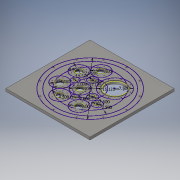
# Autodesk Inventor part: Top Plate
Saved by Autodesk Inventor 2018 (Build 220112000, 112)
## iProperties
Created: 2018-08-07
Part Number: Top Plate
Material: Stainless Steel, Austenitic
Document SubType Name: Modeling
Designer: freyja
Density: 8 g/cm^3
Appearance: Semi-Polished
Mass: 52241 g
Surface Area: 7917.75 cm^2
Volume: 6530.12 cm^3
Author: freyja
Autodesk Inventor part; units mm, degrees
ref_plane "YZ Plane" through (0, 0, 0) normal (1, 0, 0) x (0, 1, 0)
ref_plane "XZ Plane" through (0, 0, 0) normal (0, 1, 0) x (-1, 0, 0)
ref_plane "XY Plane" through (0, 0, 0) normal (0, 0, 1) x (1, 0, 0)
sketch "Sketch1" plane through (0, 0, 0) normal (0, 1, 0) x (-1, 0, 0)
  line L0 (304.8, 304.8) -> (-304.8, 304.8)
  line L1 (-304.8, 304.8) -> (-304.8, -304.8)
  line L2 (-304.8, -304.8) -> (304.8, -304.8)
  line L3 (304.8, -304.8) -> (304.8, 304.8)
  line L4 (304.8, 304.8) -> (-304.8, -304.8) construction
  line L5 (-304.8, 304.8) -> (304.8, -304.8) construction
  point P0 (0, 0)
  dimension "d0" = 609.6
  dimension "d1" = 609.6
  constraints: 12 end point, 2 midpoint, 2 parallel, 1 horizontal, 1 perpendicular
  measures "d0" distance of L2.end L1.end
  measures "d1" distance of L1.end L0.end
extrude "Extrusion1" add sketch "Sketch1" along normal blind 19.05
sketch "Sketch23" plane through (0, 19.05, 0) normal (0, 1, 0) x (1, 0, 0)
  circle A0 centre (0, 0) radius 273.05
  circle A1 centre (0, 0) radius 242.8875
  circle A2 centre (0, 0) radius 90.4875
  circle A3 centre (0, 0) radius 192.0875
  dimension "d167" = 546.1
  dimension "d168" = 485.775
  dimension "d292" = 180.975
  dimension "d293" = 384.175
  constraints: 4 centre point, 4 coincident
  measures "d167" diameter of A0
  measures "d168" diameter of A1
  measures "d292" diameter of A2
  measures "d293" diameter of A3
sketch "Sketch2" plane through (0, 19.05, 0) normal (0, 1, 0) x (1, 0, 0)
  line L0 (0, 0) -> (89.8026, 89.8026) construction
  line L1 (0, 0) -> (127, 0) construction
  circle A0 centre (89.8026, 89.8026) radius 118.745 construction
  circle A1 centre (89.8026, 89.8026) radius 66.675
  dimension "d4" = 127
  dimension "d5" = 45
  dimension "d6" = 237.49
  dimension "d7" = 133.35
  constraints: 4 end point, 2 centre point, 2 coincident, 1 equal length, 1 horizontal
  measures "d4" distance of L0.start L0.end
  measures "d5" angle of L1 L0
  measures "d6" diameter of A0
  measures "d7" diameter of A1
extrude "Extrusion2" cut sketch "Sketch2" against normal up to surface (19.05 mm away)
sketch "Sketch38" plane through (0, 19.05, 0) normal (0, 1, 0) x (1, 0, 0)
  circle A0 centre (89.8026, 89.8026) radius 66.675 projected
  circle A1 centre (89.8026, 89.8026) radius 71.247
  circle A2 centre (89.8026, 89.8026) radius 74.93
  point P0 (0, 0)
  dimension "d288" = 142.494
  dimension "d289" = 149.86
  constraints: 2 centre point, 2 coincident
  measures "d288" diameter of A1
  measures "d289" diameter of A2
extrude "Extrusion22" cut sketch "Sketch38" against normal blind 3.175 contours A2
sketch "Sketch3" plane through (0, 19.05, 0) normal (0, 1, 0) x (1, 0, 0)
  circle A0 centre (89.8026, 89.8026) radius 66.675 projected
  line L0 (89.8026, 89.8026) -> (169.5888, 56.754) construction
  line L1 (89.8026, 89.8026) -> (169.5888, 122.8511) construction
  line L2 (89.8026, 89.8026) -> (122.8511, 169.5888) construction
  line L3 (89.8026, 89.8026) -> (56.754, 169.5888) construction
  line L4 (89.8026, 89.8026) -> (10.0163, 122.8511) construction
  line L5 (89.8026, 89.8026) -> (10.0163, 56.754) construction
  line L6 (89.8026, 89.8026) -> (56.754, 10.0163) construction
  line L7 (89.8026, 89.8026) -> (122.8511, 10.0163) construction
  line L8 (89.8026, 89.8026) -> (136.7356, 70.3622) construction
  line L9 (89.8026, 89.8026) -> (140.6026, 89.8026) construction
  point P0 (0, 0)
  dimension "d10" = 86.36
  dimension "d14" = 360
  dimension "d408" = 50.8
  dimension "d409" = 22.5
  constraints: 20 end point, 2 coincident, 1 collinear, 1 equal length, 1 horizontal, 23 other
  measures "d10" distance of L0.start L0.end
  measures "d408" distance of L7.start L8.end
  measures "d409" angle of L8 L9
hole "Hole1" at (169.5888, 19.05, -56.754) at (169.5888, 19.05, -122.8511) at (122.8511, 19.05, -169.5888) at (56.754, 19.05, -169.5888) at (10.0163, 19.05, -122.8511) at (10.0163, 19.05, -56.754) at (56.754, 19.05, -10.0163) at (122.8511, 19.05, -10.0163) direction (0, -1, 0) diameter 4.9784 depth 15.24 tip angle 118 thread size "1/4-20 UNC" class "2B" standard "ANSI Unified Screw Threads"
sketch "Sketch4" plane through (0, 19.05, 0) normal (0, 1, 0) x (1, 0, 0)
  line L0 (0, 0) -> (-149.6314, -69.7743) construction
  line L1 (0, 0) -> (165.1, 0) construction
  circle A0 centre (-149.6314, -69.7743) radius 26.289
  dimension "d23" = 165.1
  dimension "d24" = 205
  dimension "d25" = 52.578
  constraints: 4 end point, 1 centre point, 1 coincident, 1 equal length, 1 horizontal
  measures "d23" distance of L0.start L0.end
  measures "d25" diameter of A0
extrude "Extrusion3" cut sketch "Sketch4" against normal blind 2.54
sketch "Sketch5" plane through (-149.6314, 16.51, 69.7743) normal (0, 1, 0) x (1, 0, 0)
  circle A0 centre (0, 0) radius 26.289 projected
  circle A1 centre (0, 0) radius 24.13
  point P0 (149.6314, 69.7743)
  dimension "d28" = 48.26
  constraints: 1 centre point, 1 coincident
  measures "d28" diameter of A1
extrude "Extrusion4" cut sketch "Sketch5" against normal up to surface (16.51 mm away) contours A1
sketch "Sketch6" plane through (0, 19.05, 0) normal (0, 1, 0) x (1, 0, 0)
  circle A0 centre (-149.6314, -69.7743) radius 24.13 construction
  line L0 (-149.6314, -69.7743) -> (-111.4983, -85.5695) construction
  line L1 (-149.6314, -69.7743) -> (-108.3564, -69.7743) construction
  line L2 (-149.6314, -69.7743) -> (-111.4983, -53.979) construction
  line L3 (-149.6314, -69.7743) -> (-133.8362, -31.6411) construction
  line L4 (-149.6314, -69.7743) -> (-165.4267, -31.6411) construction
  line L5 (-149.6314, -69.7743) -> (-187.7645, -53.979) construction
  line L6 (-149.6314, -69.7743) -> (-187.7645, -85.5695) construction
  line L7 (-149.6314, -69.7743) -> (-165.4267, -107.9074) construction
  line L8 (-149.6314, -69.7743) -> (-133.8362, -107.9074) construction
  line L9 (-149.6314, -69.7743) -> (-137.8981, -74.6344) construction
  line L10 (-149.6314, -69.7743) -> (-136.9314, -69.7743) construction
  point P0 (0, 0)
  dimension "d31" = 41.275
  dimension "d35" = 360
  dimension "d404" = 12.7
  dimension "d405" = 22.5
  constraints: 22 end point, 2 coincident, 2 horizontal, 1 collinear, 1 equal length, 23 other
  measures "d31" distance of L0.start L0.end
  measures "d404" distance of L8.start L9.end
  measures "d405" angle of L9 L10
hole "Hole2" at (-111.4983, 19.05, 53.979) at (-133.8362, 19.05, 31.6411) at (-165.4267, 19.05, 31.6411) at (-187.7645, 19.05, 53.979) at (-187.7645, 19.05, 85.5695) at (-165.4267, 19.05, 107.9074) at (-133.8362, 19.05, 107.9074) at (-111.4983, 19.05, 85.5695) direction (0, -1, 0) diameter 3.9624 depth 13.6144 tip angle 118 thread size "10-32 UNF" class "2B" standard "ANSI Unified Screw Threads"
pattern_circular "Circular Pattern1" count 3 over 180 about axis through (0, -10, 0) along (0, 1, 0) of "Extrusion4", "Extrusion3", "Hole2" both ways yes
sketch "Sketch7" plane through (0, 19.05, 0) normal (0, 1, 0) x (1, 0, 0)
  line L0 (0, 0) -> (-43.7065, 62.4194) construction
  line L1 (0, 0) -> (76.2, 0) construction
  circle A0 centre (-43.7065, 62.4194) radius 13.208
  dimension "d44" = 76.2
  dimension "d45" = 125
  dimension "d46" = 26.416
  constraints: 4 end point, 1 centre point, 1 coincident, 1 equal length, 1 horizontal
  measures "d44" distance of L0.start L0.end
  measures "d45" angle of L1 L0
  measures "d46" diameter of A0
extrude "Extrusion5" cut sketch "Sketch7" against normal blind 2.54
sketch "Sketch8" plane through (0, 19.05, 0) normal (0, 1, 0) x (1, 0, 0)
  circle A0 centre (-43.7065, 62.4194) radius 13.208 projected
  circle A1 centre (-43.7065, 62.4194) radius 11.43
  point P0 (0, 0)
  dimension "d49" = 22.86
  constraints: 1 centre point, 1 coincident
  measures "d49" diameter of A1
extrude "Extrusion6" cut sketch "Sketch8" against normal up to surface (19.05 mm away) contours A1
sketch "Sketch9" plane through (0, 19.05, 0) normal (0, 1, 0) x (1, 0, 0)
  circle A0 centre (-43.7065, 62.4194) radius 13.208 projected
  line L0 (-43.7065, 62.4194) -> (-19.7035, 62.4194) construction
  line L1 (-43.7065, 62.4194) -> (-19.7035, 62.4194) construction
  line L2 (-43.7065, 62.4194) -> (-31.705, 83.2066) construction
  line L3 (-43.7065, 62.4194) -> (-55.708, 83.2066) construction
  line L4 (-43.7065, 62.4194) -> (-67.7095, 62.4194) construction
  line L5 (-43.7065, 62.4194) -> (-55.708, 41.6322) construction
  line L6 (-43.7065, 62.4194) -> (-31.705, 41.6322) construction
  point P0 (0, 0)
  dimension "d52" = 24.003
  dimension "d53" = 0
  dimension "d56" = 360
  constraints: 14 end point, 2 coincident, 2 horizontal, 1 collinear, 17 other
  measures "d52" distance of L0.start L0.end
  measures "d53" distance between parallel lines of L0 L1
hole "Hole3" at (-19.7035, 19.05, -62.4194) at (-31.705, 19.05, -83.2066) at (-55.708, 19.05, -83.2066) at (-67.7095, 19.05, -62.4194) at (-55.708, 19.05, -41.6322) at (-31.705, 19.05, -41.6322) direction (0, -1, 0) diameter 3.9624 depth 13.6144 tip angle 118 thread size "10-32 UNF" class "2B" standard "ANSI Unified Screw Threads"
sketch "Sketch26" plane through (0, 19.05, 0) normal (0, 1, 0) x (1, 0, 0)
  line L0 (0, 0) -> (-107.95, 0) construction
  line L1 (0, 0) -> (107.95, 0) construction
  circle A0 centre (-107.95, 0) radius 8.636
  dimension "d185" = 107.95
  dimension "d186" = 180
  dimension "d187" = 17.272
  constraints: 4 end point, 1 centre point, 1 coincident, 1 collinear, 1 horizontal
  measures "d185" distance of L0.start L0.end
  measures "d186" angle of L0 L1
  measures "d187" diameter of A0
extrude "Extrusion16" cut sketch "Sketch26" against normal blind 2.54
sketch "Sketch27" plane through (0, 19.05, 0) normal (0, 1, 0) x (1, 0, 0)
  circle A0 centre (-107.95, 0) radius 8.636 projected
  circle A1 centre (-107.95, 0) radius 6.35
  point P0 (0, 0)
  dimension "d190" = 12.7
  constraints: 1 centre point, 1 coincident
  measures "d190" diameter of A1
extrude "Extrusion17" cut sketch "Sketch27" against normal up to surface (19.05 mm away) contours A1
sketch "Sketch28" plane through (0, 19.05, 0) normal (0, 1, 0) x (1, 0, 0)
  circle A0 centre (-107.95, 0) radius 8.636 projected
  line L0 (-107.95, 0) -> (-127, 0) construction
  line L1 (-107.95, 0) -> (-88.9, 0) construction
  line L2 (-107.95, 0) -> (-117.475, -16.4978) construction
  line L3 (-107.95, 0) -> (-98.425, -16.4978) construction
  line L4 (-107.95, 0) -> (-88.9, 0) construction
  line L5 (-107.95, 0) -> (-98.425, 16.4978) construction
  line L6 (-107.95, 0) -> (-117.475, 16.4978) construction
  point P0 (0, 0)
  dimension "d193" = 19.05
  dimension "d194" = 180
  dimension "d204" = 360
  constraints: 14 end point, 2 coincident, 2 horizontal, 1 collinear, 17 other
  measures "d193" distance of L0.start L0.end
  measures "d194" angle of L0 L1
hole "Hole9" at (-127, 19.05, 0) at (-117.475, 19.05, -16.4978) at (-98.425, 19.05, -16.4978) at (-88.9, 19.05, 0) at (-98.425, 19.05, 16.4978) at (-117.475, 19.05, 16.4978) direction (0, -1, 0) diameter 3.9624 depth 13.6144 tip angle 118 thread size "10-32 UNF" class "2B" standard "ANSI Unified Screw Threads"
pattern_circular "Circular Pattern6" count 2 over 90 about axis through (0, -10, 0) along (0, 1, 0) of "Extrusion16", "Extrusion17", "Hole9"
sketch "Sketch30" plane through (0, 19.05, 0) normal (0, 1, 0) x (1, 0, 0)
  line L0 (0, 0) -> (-69.7743, -149.6314) construction
  line L1 (0, 0) -> (165.1, 0) construction
  circle A0 centre (-69.7743, -149.6314) radius 26.289
  dimension "d221" = 165.1
  dimension "d222" = 115
  dimension "d223" = 52.578
  constraints: 4 end point, 1 centre point, 1 coincident, 1 equal length, 1 horizontal
  measures "d221" distance of L0.start L0.end
  measures "d222" angle of L0 L1
  measures "d223" diameter of A0
extrude "Extrusion18" cut sketch "Sketch30" against normal blind 2.54
sketch "Sketch31" plane through (0, 19.05, 0) normal (0, 1, 0) x (1, 0, 0)
  circle A0 centre (-69.7743, -149.6314) radius 26.289 projected
  circle A1 centre (-69.7743, -149.6314) radius 24.13
  point P0 (0, 0)
  dimension "d226" = 48.26
  constraints: 1 centre point, 1 coincident
  measures "d226" diameter of A1
extrude "Extrusion19" cut sketch "Sketch31" against normal up to surface (19.05 mm away) contours A1
sketch "Sketch32" plane through (0, 19.05, 0) normal (0, 1, 0) x (1, 0, 0)
  circle A0 centre (-69.7743, -149.6314) radius 26.289 construction
  line L0 (-69.7743, -149.6314) -> (-107.9074, -133.8362) construction
  line L1 (-69.7743, -149.6314) -> (-107.9074, -165.4267) construction
  line L2 (-69.7743, -149.6314) -> (-85.5695, -187.7645) construction
  line L3 (-69.7743, -149.6314) -> (-53.979, -187.7645) construction
  line L4 (-69.7743, -149.6314) -> (-31.6411, -165.4267) construction
  line L5 (-69.7743, -149.6314) -> (-31.6411, -133.8362) construction
  line L6 (-69.7743, -149.6314) -> (-53.979, -111.4983) construction
  line L7 (-69.7743, -149.6314) -> (-85.5695, -111.4983) construction
  line L8 (-69.7743, -149.6314) -> (-58.041, -154.4915) construction
  line L9 (-69.7743, -149.6314) -> (-57.0743, -149.6314) construction
  point P0 (0, 0)
  dimension "d229" = 41.275
  dimension "d232" = 360
  dimension "d406" = 12.7
  dimension "d407" = 22.5
  constraints: 20 end point, 2 coincident, 1 collinear, 1 equal length, 1 horizontal, 23 other
  measures "d229" distance of L0.start L0.end
  measures "d406" distance of L7.start L8.end
  measures "d407" angle of L8 L9
hole "Hole10" at (-85.5695, 19.05, 111.4983) at (-107.9074, 19.05, 133.8362) at (-53.979, 19.05, 111.4983) at (-31.6411, 19.05, 133.8362) at (-31.6411, 19.05, 165.4267) at (-53.979, 19.05, 187.7645) at (-85.5695, 19.05, 187.7645) at (-107.9074, 19.05, 165.4267) direction (0, -1, 0) diameter 3.9624 depth 13.6144 tip angle 118 thread size "10-32 UNF" class "2B" standard "ANSI Unified Screw Threads"
pattern_circular "Circular Pattern7" count 2 over 90 about axis through (0, -10, 0) along (0, -1, 0) of "Extrusion18", "Extrusion19", "Hole10" both ways yes
sketch "Sketch37" plane through (0, 19.05, 0) normal (0, 1, 0) x (1, 0, 0)
  line L0 (0, 0) -> (-264.16, 0)
  dimension "d277" = 264.16
  constraints: 2 end point, 1 horizontal
  measures "d277" distance of L0.start L0.end
hole "Hole13" at (-264.16, 19.05, 0) direction (0, -1, 0) diameter 8.9916 depth 21.1074 tip angle 118 clearance for "Socket Head Cap Screw" size "M8" standard "Ansi Metric M Profile"
pattern_circular "Circular Pattern9" count 12 over 360 about axis through (0, -10, 0) along (0, 1, 0) of "Hole13"
sketch "Sketch39" plane through (0, 19.05, 0) normal (0, 1, 0) x (1, 0, 0)
  line L0 (0, 0) -> (-35.921, -35.921) construction
  line L1 (0, 0) -> (50.8, 0) construction
  circle A0 centre (-35.921, -35.921) radius 26.289
  dimension "d294" = 50.8
  dimension "d295" = 135
  dimension "d296" = 52.578
  constraints: 4 end point, 1 centre point, 1 coincident, 1 equal length, 1 horizontal
  measures "d294" distance of L0.start L0.end
  measures "d295" angle of L0 L1
  measures "d296" diameter of A0
extrude "Extrusion23" cut sketch "Sketch39" against normal blind 2.54
sketch "Sketch40" plane through (0, 19.05, 0) normal (0, 1, 0) x (1, 0, 0)
  circle A0 centre (-35.921, -35.921) radius 26.289 projected
  circle A1 centre (-35.921, -35.921) radius 24.13
  point P0 (0, 0)
  dimension "d299" = 48.26
  constraints: 1 centre point, 1 coincident
  measures "d299" diameter of A1
extrude "Extrusion24" cut sketch "Sketch40" against normal up to surface (19.05 mm away) contours A1
sketch "Sketch41" plane through (0, 19.05, 0) normal (0, 1, 0) x (1, 0, 0)
  circle A0 centre (-35.921, -35.921) radius 24.13 projected
  line L0 (-35.921, -35.921) -> (5.354, -35.921) construction
  line L1 (-35.921, -35.921) -> (5.354, -35.921) construction
  line L2 (-35.921, -35.921) -> (-6.7352, -6.7352) construction
  line L3 (-35.921, -35.921) -> (-35.921, 5.354) construction
  line L4 (-35.921, -35.921) -> (-65.1069, -6.7352) construction
  line L5 (-35.921, -35.921) -> (-77.196, -35.921) construction
  line L6 (-35.921, -35.921) -> (-65.1069, -65.1069) construction
  line L7 (-35.921, -35.921) -> (-35.921, -77.196) construction
  line L8 (-35.921, -35.921) -> (-6.7352, -65.1069) construction
  point P0 (0, 0)
  dimension "d302" = 41.275
  dimension "d303" = 0
  dimension "d306" = 360
  constraints: 18 end point, 2 coincident, 2 horizontal, 1 collinear, 23 other
  measures "d302" distance of L0.start L0.end
  measures "d303" distance between parallel lines of L0 L1
hole "Hole14" at (-6.7352, 19.05, 65.1069) at (5.354, 19.05, 35.921) at (-6.7352, 19.05, 6.7352) at (-35.921, 19.05, -5.354) at (-65.1069, 19.05, 6.7352) at (-77.196, 19.05, 35.921) at (-65.1069, 19.05, 65.1069) at (-35.921, 19.05, 77.196) direction (0, -1, 0) diameter 3.9624 depth 13.6144 tip angle 118 thread size "10-32 UNF" class "2B" standard "ANSI Unified Screw Threads"
pattern_circular "Circular Pattern11" count 2 over 200 about axis through (0, -10, 0) along (0, 1, 0) of "Extrusion5", "Extrusion6", "Hole3"
sketch "Sketch45" plane through (0, 19.05, 0) normal (0, 1, 0) x (1, 0, 0)
  line L0 (0, 0) -> (123.1835, -71.12) construction
  line L1 (0, 0) -> (142.24, 0) construction
  circle A0 centre (123.1835, -71.12) radius 13.208
  dimension "d384" = 165.1
  dimension "d385" = 0
  dimension "d388" = 25.4
  dimension "d389" = 45
  dimension "d392" = 360
  dimension "d349" = 142.24
  dimension "d350" = 30
  dimension "d351" = 26.416
  constraints: 4 end point, 1 centre point, 1 coincident, 1 equal length, 1 horizontal
  measures "d349" distance of L0.start L0.end
  measures "d350" angle of L0 L1
  measures "d351" diameter of A0
extrude "Extrusion27" cut sketch "Sketch45" against normal blind 2.54
sketch "Sketch46" plane through (0, 19.05, 0) normal (0, 1, 0) x (1, 0, 0)
  circle A0 centre (123.1835, -71.12) radius 13.208 projected
  circle A1 centre (123.1835, -71.12) radius 11.43
  point P0 (0, 0)
  dimension "d354" = 22.86
  constraints: 1 centre point, 1 coincident
  measures "d354" diameter of A1
extrude "Extrusion28" cut sketch "Sketch46" against normal up to surface (19.05 mm away) contours A1
sketch "Sketch47" plane through (0, 19.05, 0) normal (0, 1, 0) x (1, 0, 0)
  circle A0 centre (123.1835, -71.12) radius 11.43 projected
  line L0 (123.1835, -71.12) -> (144.0806, -59.055) construction
  line L1 (123.1835, -71.12) -> (147.3135, -71.12) construction
  line L2 (123.1835, -71.12) -> (123.1835, -46.99) construction
  line L3 (123.1835, -71.12) -> (102.2863, -59.055) construction
  line L4 (123.1835, -71.12) -> (102.2863, -83.185) construction
  line L5 (123.1835, -71.12) -> (123.1835, -95.25) construction
  line L6 (123.1835, -71.12) -> (144.0806, -83.185) construction
  point P0 (0, 0)
  dimension "d357" = 24.13
  dimension "d358" = 30
  dimension "d361" = 360
  constraints: 14 end point, 2 coincident, 1 equal length, 1 horizontal, 17 other
  measures "d357" distance of L0.start L0.end
  measures "d358" angle of L1 L0
hole "Hole16" at (144.0806, 19.05, 83.185) at (123.1835, 19.05, 95.25) at (102.2863, 19.05, 83.185) at (102.2863, 19.05, 59.055) at (123.1835, 19.05, 46.99) at (144.0806, 19.05, 59.055) direction (0, -1, 0) diameter 3.9624 depth 13.6144 tip angle 118 thread size "10-32 UNF" class "2B" standard "ANSI Unified Screw Threads"
sketch "Sketch48" plane through (0, 0, 0) normal (0, -1, 0) x (1, 0, 0)
  circle A0 centre (-35.921, 35.921) radius 24.13 projected
  line L0 (-35.921, 35.921) -> (2.2121, 51.7163) construction
  line L1 (-35.921, 35.921) -> (5.354, 35.921) construction
  line L2 (-35.921, 35.921) -> (-20.1258, 74.0542) construction
  line L3 (-35.921, 35.921) -> (-51.7163, 74.0542) construction
  line L4 (-35.921, 35.921) -> (-74.0542, 51.7163) construction
  line L5 (-35.921, 35.921) -> (-74.0542, 20.1258) construction
  line L6 (-35.921, 35.921) -> (-51.7163, -2.2121) construction
  line L7 (-35.921, 35.921) -> (-20.1258, -2.2121) construction
  line L8 (-35.921, 35.921) -> (2.2121, 20.1258) construction
  point P0 (0, 0)
  dimension "d371" = 41.275
  dimension "d372" = 22.5
  dimension "d375" = 360
  constraints: 18 end point, 2 coincident, 1 equal length, 1 horizontal, 23 other
  measures "d371" distance of L0.start L0.end
  measures "d372" angle of L1 L0
hole "Hole17" at (-20.1258, 0, 74.0542) at (-51.7163, 0, 74.0542) at (-74.0542, 0, 51.7163) at (-74.0542, 0, 20.1258) at (-51.7163, 0, -2.2121) at (-20.1258, 0, -2.2121) at (2.2121, 0, 20.1258) at (2.2121, 0, 51.7163) direction (0, 1, 0) diameter 3.9624 depth 13.6144 tip angle 118 thread size "10-32 UNF" class "2B" standard "ANSI Unified Screw Threads"
sketch "Sketch49" plane through (0, 0, 0) normal (0, -1, 0) x (1, 0, 0)
  line L0 (0, 0) -> (165.1, 0) construction
  line L1 (0, 0) -> (165.1, 0) construction
  line L2 (165.1, 0) -> (152.4, 0) construction
  line L3 (165.1, 0) -> (183.0605, 17.9605) construction
  line L4 (165.1, 0) -> (190.5, 0) construction
  line L5 (165.1, 0) -> (147.1395, 17.9605) construction
  line L6 (165.1, 0) -> (147.1395, -17.9605) construction
  line L7 (165.1, 0) -> (183.0605, -17.9605) construction
  dimension "d384" = 165.1
  dimension "d385" = 0
  dimension "d388" = 25.4
  dimension "d389" = 45
  dimension "d392" = 360
  constraints: 16 end point, 3 horizontal, 2 equal length, 13 other
  measures "d384" distance of L0.start L0.end
  measures "d385" distance between parallel lines of L1 L0
  measures "d388" distance of L1.end L3.end
  measures "d389" angle of L4 L3
hole "Hole18" at (183.0605, 0, -17.9605) at (147.1395, 0, -17.9605) at (147.1395, 0, 17.9605) at (183.0605, 0, 17.9605) direction (0, 1, 0) diameter 4.3434 depth 16.256 tip angle 118 thread size "12-24 UNC" class "2B" standard "ANSI Unified Screw Threads"
pattern_circular "Circular Pattern12" count 4 over 360 about axis through (0, -10, 0) along (0, 1, 0) of "Hole18"
sketch "Sketch25" plane through (0, 19.05, 0) normal (0, 1, 0) x (1, 0, 0)
  circle A0 centre (-149.6314, -69.7743) radius 26.289 projected
  circle A1 centre (-149.6314, -69.7743) radius 57.15
  circle A2 centre (89.8026, 89.8026) radius 66.675 projected
  circle A3 centre (89.8026, 89.8026) radius 95.25
  circle A4 centre (-43.7065, 62.4194) radius 11.43 projected
  circle A5 centre (-43.7065, 62.4194) radius 31.75
  circle A6 centre (-107.95, 0) radius 6.35 projected
  circle A7 centre (-107.95, 0) radius 25.4
  circle A8 centre (-69.7743, -149.6314) radius 24.13 projected
  circle A9 centre (-69.7743, -149.6314) radius 57.15
  circle A10 centre (-69.7743, 149.6314) radius 24.13 projected
  circle A11 centre (-69.7743, 149.6314) radius 57.15
  circle A12 centre (-149.6314, 69.7743) radius 24.13 projected
  circle A13 centre (-149.6314, 69.7743) radius 57.15
  circle A14 centre (-35.921, -35.921) radius 24.13 projected
  circle A15 centre (-35.921, -35.921) radius 57.15
  circle A16 centre (62.4194, -43.7065) radius 13.208 projected
  circle A17 centre (62.4194, -43.7065) radius 31.75
  circle A18 centre (69.7743, -149.6314) radius 26.289 projected
  circle A19 centre (69.7743, -149.6314) radius 57.15
  circle A20 centre (0, -107.95) radius 6.35 projected
  circle A21 centre (0, -107.95) radius 25.4
  circle A22 centre (123.1835, -71.12) radius 11.43 projected
  circle A23 centre (123.1835, -71.12) radius 31.75
  point P0 (0, 0)
  dimension "d206" = 114.3
  dimension "d207" = 190.5
  dimension "d208" = 63.5
  dimension "d209" = 50.8
  dimension "d241" = 114.3
  dimension "d246" = 114.3
  dimension "d318" = 114.3
  dimension "d320" = 114.3
  dimension "d324" = 63.5
  dimension "d325" = 114.3
  dimension "d326" = 50.8
  dimension "d370" = 63.5
  constraints: 12 centre point, 12 coincident
  measures "d206" diameter of A1
  measures "d207" diameter of A3
  measures "d208" diameter of A5
  measures "d209" diameter of A7
  measures "d241" diameter of A9
  measures "d246" diameter of A11
  measures "d318" diameter of A13
  measures "d320" diameter of A15
  measures "d324" diameter of A17
  measures "d325" diameter of A19
  measures "d326" diameter of A21
  measures "d370" diameter of A23
body "Solid1"
